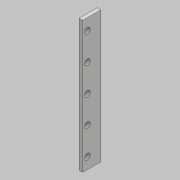
# Autodesk Inventor part: exercise3-12
Saved by Autodesk Inventor 2018 (Build 220112000, 112)
## iProperties
Created: 2020-09-23
Part Number: exercise3-12
Material: 一般
Document SubType Name: Modeling
Designer: 王鼎鈞
Density: 1 g/cm^3
Appearance: 預設
Author: 王鼎鈞
Autodesk Inventor part; units mm, degrees
ref_plane "YZ Plane" through (0, 0, 0) normal (1, 0, 0) x (0, 1, 0)
ref_plane "XZ Plane" through (0, 0, 0) normal (0, 1, 0) x (-1, 0, 0)
ref_plane "XY Plane" through (0, 0, 0) normal (0, 0, 1) x (1, 0, 0)
sketch "草圖1" plane through (0, 0, 0) normal (1, 0, 0) x (0, 1, 0)
  line L0 (0, 0) -> (80, 0)
  line L1 (80, 0) -> (80, -580)
  line L2 (80, -580) -> (0, -580)
  line L3 (0, -580) -> (0, 0)
  dimension "d0" = 80
  dimension "d1" = 580
  constraints: 8 end point, 2 parallel, 1 horizontal, 1 perpendicular
  measures "d0" distance of L1.end L2.end
  measures "d1" distance of L0.end L1.end
extrude "擠出1" add sketch "草圖1" along normal blind 16
sketch "草圖2" plane through (16, 0, 0) normal (1, 0, 0) x (0, 0, -1)
  line L0 (0, 80) -> (0, 0) projected
  line L1 (0, 0) -> (580, 0) projected
  point P0 (50, 20)
  point P1 (170, 20)
  point P2 (290, 20)
  point P3 (410, 20)
  point P4 (530, 20)
  dimension "d4" = 50
  dimension "d5" = 20
  dimension "d6" = 120
  dimension "d7" = 120
  dimension "d8" = 120
  dimension "d9" = 120
  dimension "d10" = 20
  dimension "d11" = 20
  dimension "d12" = 20
  dimension "d13" = 20
  measures "d4" distance from line of L0 point (50, 20)
  measures "d5" distance from line of L1 point (50, 20)
  measures "d6" distance of point (50, 20) point (170, 20)
  measures "d7" distance of point (170, 20) point (290, 20)
  measures "d8" distance of point (290, 20) point (410, 20)
  measures "d9" distance of point (410, 20) point (530, 20)
  measures "d10" distance from line of L1 point (170, 20)
  measures "d11" distance from line of L1 point (290, 20)
  measures "d12" distance from line of L1 point (410, 20)
  measures "d13" distance from line of L1 point (530, 20)
hole "孔1" at (16, 20, -50) at (16, 20, -170) at (16, 20, -290) at (16, 20, -410) at (16, 20, -530) direction (-1, 0, 0) diameter 25.2 end through all
